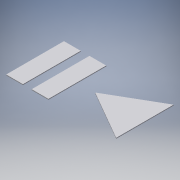
# Autodesk Inventor part: Pause
Saved by Autodesk Inventor 2018 (Build 220112000, 112)
## iProperties
Created: 2022-03-18
Part Number: Pause
Material: Generisch
Document SubType Name: Modeling
Designer: Markus
Density: 1 g/cm^3
Appearance: Vorgabe
Author: Markus
Autodesk Inventor part; units mm, degrees
ref_plane "YZ Plane" through (0, 0, 0) normal (1, 0, 0) x (0, 1, 0)
ref_plane "XZ Plane" through (0, 0, 0) normal (0, 1, 0) x (-1, 0, 0)
ref_plane "XY Plane" through (0, 0, 0) normal (0, 0, 1) x (1, 0, 0)
sketch "Skizze1" plane through (0, 0, 0) normal (0, 0, 1) x (1, 0, 0)
  line L0 (-9.1332, 7) -> (-9.1332, -7) projected
  line L1 (-9.1332, -7) -> (-13.2665, -7) projected
  line L2 (-13.2665, -7) -> (-13.2665, 7) projected
  line L3 (-13.2665, 7) -> (-9.1332, 7) projected
  line L4 (-3, 7) -> (-3, -7) projected
  line L5 (-3, -7) -> (-7.1332, -7) projected
  line L6 (-7.1332, -7) -> (-7.1332, 7) projected
  line L7 (-7.1332, 7) -> (-3, 7) projected
  line L8 (1.1421, 0) -> (13.2665, 7) projected
  line L9 (13.2665, 7) -> (13.2665, -7) projected
  line L10 (13.2665, -7) -> (1.1421, 0) projected
  circle A0 centre (0, 0) radius 18.6906 projected
  line L11 (-3.05, -6.95) -> (-3.05, 6.95)
  line L12 (-3.05, 6.95) -> (-7.0832, 6.95)
  line L13 (-7.0832, 6.95) -> (-7.0832, -6.95)
  line L14 (-7.0832, -6.95) -> (-3.05, -6.95)
  line L15 (-9.1832, -6.95) -> (-9.1832, 6.95)
  line L16 (-9.1832, 6.95) -> (-13.2165, 6.95)
  line L17 (-13.2165, 6.95) -> (-13.2165, -6.95)
  line L18 (-13.2165, -6.95) -> (-9.1832, -6.95)
  line L19 (13.2165, 6.9134) -> (1.2421, 0)
  line L20 (1.2421, 0) -> (13.2165, -6.9134)
  line L21 (13.2165, -6.9134) -> (13.2165, 6.9134)
  point P0 (0, 0)
  point P1 (-1.0928, 10.1918)
  dimension "d0" = 0.05
  dimension "d1" = 0.05
  dimension "d2" = 0.05
  constraints: 22 end point, 9 other
  measures "d0" distance between parallel lines of L4 L11
  measures "d1" distance between parallel lines of L0 L15
  measures "d2" distance between parallel lines of L8 L19
extrude "Extrusion1" add sketch "Skizze1" against normal blind 0.2 contours L14 L13 L12 L11 | L18 L17 L16 L15 | L21 L20 L19
